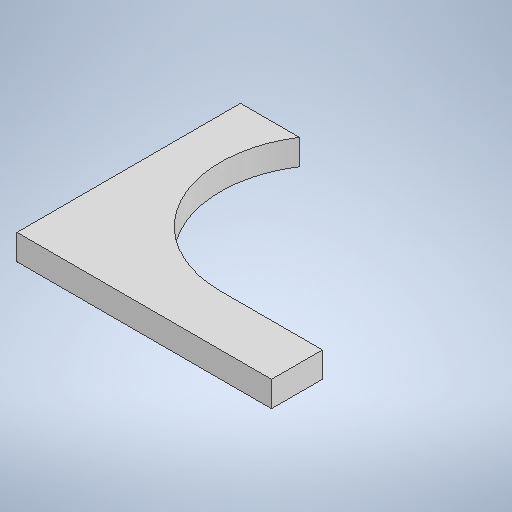
# Autodesk Inventor part: WoodBoundaryV1
Saved by Autodesk Inventor 2025.1 (Build 291241000, 241)
## iProperties
Created: 2025-10-12
Part Number: WoodBoundaryV1
Material: Generic
Document SubType Name: Modeling
Designer: jonas
Density: 1 g/cm^3
Appearance: Default
Author: jonas
Autodesk Inventor part; units mm, degrees
ref_plane "YZ Plane" through (0, 0, 0) normal (1, 0, 0) x (0, 1, 0)
ref_plane "XZ Plane" through (0, 0, 0) normal (0, 1, 0) x (-1, 0, 0)
ref_plane "XY Plane" through (0, 0, 0) normal (0, 0, 1) x (1, 0, 0)
sketch "Sketch1" plane through (0, 0, 0) normal (0, 1, 0) x (-1, 0, 0)
  line L0 (0, -151.455) -> (0, 151.455) construction
  line L1 (30.6851, 0) -> (-30.6851, 0) construction
  arc A0 (184.1467, -119.55) -> (0, 219.55) centre (0, 0) ccw
  line L2 (0, 219.55) -> (-200, 219.55)
  line L3 (-200, 219.55) -> (-200, 319.55)
  line L4 (-200, 319.55) -> (300, 319.55)
  line L5 (300, 319.55) -> (300, -119.55)
  line L6 (300, -119.55) -> (184.1467, -119.55)
  dimension "d0" = 439.1
  dimension "d1" = 200
  dimension "d3" = 100
  dimension "d4" = 119.55
  dimension "d5" = 300
  constraints: 14 end point, 3 perpendicular, 2 coincident, 2 horizontal, 2 midpoint, 2 point on circle, 2 vertical, 1 centre point, 1 tangent
  measures "d0" diameter of A0
  measures "d1" distance of L2.start L2.end
  measures "d3" distance of L2.end L3.end
  measures "d4" distance from line of point (0, 0) L6
  measures "d5" distance from line of point (0, 0) L5
extrude "Extrusion1" add sketch "Sketch1" along normal blind 50
body "Solid1"
